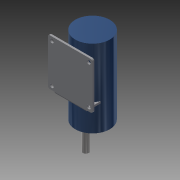
# Autodesk Inventor part: Moteur
Saved by Autodesk Inventor 2016 (Build 200138000, 138)
## iProperties
Created: 2015-04-27
Part Number: Moteur
Material: Générique
Document SubType Name: Modeling
Designer: Logan
Density: 1 g/cm^3
Appearance: Par défaut
Author: Logan
Autodesk Inventor part; units mm, degrees
ref_plane "YZ Plane" through (0, 0, 0) normal (1, 0, 0) x (0, 1, 0)
ref_plane "XZ Plane" through (0, 0, 0) normal (0, 1, 0) x (-1, 0, 0)
sketch "Esquisse1" plane through (0, 0, 0) normal (0, 0, 1) x (1, 0, 0)
  arc A0 (-1.6583, -4.5) -> (1.6583, -4.5) centre (0, -7) ccw
  line L0 (1.6583, -4.5) -> (-1.6583, -4.5)
  point P0 (0, 0)
  dimension "d2" = 6
  dimension "d4" = 7
  dimension "d11" = 0.5
  constraints: 2 end point, 2 point on circle, 1 centre point, 1 horizontal
  measures "d2" diameter of A0
  measures "d4" distance of point (0, 0) A0.centre
  measures "d11" distance edge to line of A0 L0
extrude "Extrusion1" add sketch "Esquisse1" against normal blind 25
sketch "Esquisse2" plane through (0, -7, 0) normal (0, 0, 1) x (1, 0, 0)
  circle A0 centre (0, 7) radius 17.75
  dimension "d8" = 35.5
  constraints: 1 centre point, 1 coincident
  measures "d8" diameter of A0
extrude "Extrusion2" add sketch "Esquisse2" along normal blind 80
ref_plane "Plan de construction1" through (0, 0, 26) normal (0, 0, -1) x (-1, 0, 0)
sketch "Esquisse3" plane through (0, 0, 26) normal (0, 0, -1) x (-1, 0, 0)
  circle A0 centre (0, 0) radius 17.75 projected
  line L0 (1.6583, -4.5) -> (-1.6583, -4.5) projected
  arc A1 (-1.6583, -4.5) -> (1.6583, -4.5) centre (0, -7) ccw projected
  line L1 (-16, -7.6852) -> (-16, -21)
  line L2 (-16, -21) -> (0, -21)
  line L3 (16, -7.6852) -> (16, -21)
  line L4 (16, -21) -> (0, -21)
  arc A2 (-16, -7.6852) -> (16, -7.6852) centre (0, 0) ccw
  circle A3 centre (0, 0) radius 17.75 projected
  line L5 (-3, -7) -> (0, -7)
  line L6 (0, -4.5) -> (0, -7)
  dimension "d14" = 16
  constraints: 12 end point, 5 point on circle, 2 concentric, 2 vertical, 1 centre point, 1 horizontal, 1 midpoint, 1 perpendicular
  measures "d14" distance from line of point (0, 0) L1
extrude "Extrusion3" add sketch "Esquisse3" against normal blind 2 contours A0 L3 L4 L2 L1
sketch "Esquisse4" plane through (0, 0, 28) normal (0, 0, 1) x (1, 0, 0)
  line L0 (-23, -21) -> (23, -21)
  line L1 (23, -21) -> (23, -23)
  line L2 (23, -23) -> (-23, -23)
  line L3 (-23, -23) -> (-23, -21)
  point P0 (0, 0)
  dimension "d18" = 2
  dimension "d19" = 46
  constraints: 8 end point, 2 parallel, 1 horizontal, 1 perpendicular, 1 point on line
  measures "d18" distance of L3.end L2.end
  measures "d19" distance of L0.start L0.end
extrude "Extrusion4" add sketch "Esquisse4" along normal blind 48
fillet "Congé1" radius 2 4 edges at (-23, -22, 28) (-23, -22, 76) (23, -22, 76) (23, -22, 28)
sketch "Esquisse5" plane through (16, -21, 26) normal (1, 0, 0) x (0, 0, -1)
  arc A0 (-2, -2) -> (0, 0) centre (-2, 0) ccw
  line L0 (-2, 0) -> (-2, -2)
  line L1 (-2, -2) -> (-2, 0) projected
  line L2 (-2, 0) -> (0, 0)
  line L3 (0, 0) -> (-2, 0) projected
  point P0 (26, 21)
  constraints: 4 end point, 2 collinear, 2 point on circle, 1 centre point
extrude "Extrusion5" add sketch "Esquisse5" against normal blind 32
fillet "Congé2" radius 2 1 edges at (0, -21, 28)
sketch "Esquisse6" plane through (-21, -21, 28) normal (0, 1, 0) x (1, 0, 0)
  line L0 (40, -4) -> (2, -4)
  line L1 (2, -4) -> (2, -44)
  line L2 (2, -44) -> (40, -44)
  line L3 (40, -44) -> (40, -4)
  line L4 (44, -2) -> (44, -46) projected
  line L5 (42, 0) -> (37, 0) projected
  line L6 (42, -48) -> (0, -48) projected
  line L7 (-2, -2) -> (-2, -46) projected
  point P0 (21, 28)
  dimension "d28" = 4
  dimension "d29" = 4
  dimension "d30" = 4
  dimension "d31" = 4
  constraints: 8 end point, 2 parallel, 1 horizontal, 1 perpendicular
  measures "d28" distance between parallel lines of L4 L3
  measures "d29" distance between parallel lines of L5 L0
  measures "d30" distance between parallel lines of L6 L2
  measures "d31" distance between parallel lines of L7 L1
hole "Perçage1" at (-19, -21, 32) at (-19, -21, 72) at (19, -21, 72) at (19, -21, 32) direction (0, -1, 0) diameter 4 end through all
